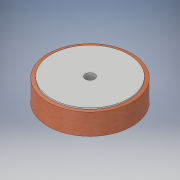
# Autodesk Inventor part: Rad
Saved by Autodesk Inventor 2017 (Build 210142000, 142)
## iProperties
Part Number: Rad
Material: Generisch
Document SubType Name: Modeling
Designer: Dima
Density: 1 g/cm^3
Appearance: Vorgabe
Author: Dima
Autodesk Inventor part; units mm, degrees
ref_plane "YZ Plane" through (0, 0, 0) normal (1, 0, 0) x (0, 1, 0)
ref_plane "XZ Plane" through (0, 0, 0) normal (0, 1, 0) x (-1, 0, 0)
ref_plane "XY Plane" through (0, 0, 0) normal (0, 0, 1) x (1, 0, 0)
sketch "Skizze1" plane through (0, 0, 0) normal (0, 1, 0) x (-1, 0, 0)
  line L0 (4, 10) -> (33, 10)
  line L1 (33, 10) -> (33, 9)
  line L2 (33, 9) -> (31, 9)
  line L3 (31, 9) -> (31, -9)
  line L4 (31, -9) -> (33, -9)
  line L5 (33, -9) -> (33, -10)
  line L6 (33, -10) -> (11.5, -10)
  line L7 (11.5, -10) -> (11.5, -5.5)
  line L8 (11.5, -5.5) -> (4, -5.5)
  line L9 (4, -5.5) -> (4, 10)
  line L10 (0, -14) -> (0, 14) construction
  line L11 (39.6, 0) -> (-6.6, 0) construction
  point P0 (0, 0)
  point P1 (31, 0)
  dimension "d0" = 4
  dimension "d1" = 2
  dimension "d2" = 33
  dimension "d3" = 18
  dimension "d4" = 20
  dimension "d5" = 4.5
  dimension "d6" = 11.5
  constraints: 20 end point, 8 perpendicular, 2 point on line, 1 horizontal, 1 horizontal alignment, 1 midpoint, 1 symmetric about line
  measures "d0" distance between parallel lines of L10 L9
  measures "d1" distance of L3.end L4.end
  measures "d2" distance from line of L10 L5.end
  measures "d3" distance of L2.end L3.end
  measures "d4" distance of L0.end L5.end
  measures "d5" distance of L6.end L7.end
  measures "d6" distance from line of L10 L6.end
revolve "Umdrehung1" add sketch "Skizze1" angle 360 about axis through (0, 0, -10) along (0, 0, 1)
sketch "Skizze2" plane through (0, 0, 0) normal (1, 0, 0) x (0, 1, 0)
  line L0 (-33, -9) -> (33, -9) construction
  line L1 (31, 9) -> (31, -9) construction
  line L2 (-33, 9) -> (33, 9) construction
  line L3 (36, -9) -> (31, -9)
  line L4 (31, -9) -> (31, 9)
  line L5 (31, 9) -> (36, 9)
  line L6 (36, 9) -> (36, -9)
  line L7 (0, -14) -> (0, 14) projected
  point P0 (0, 0)
  dimension "d8" = 5
  constraints: 8 end point, 2 parallel, 1 horizontal, 1 perpendicular
  measures "d8" distance of L3.start L1.end
revolve "Umdrehung2" add sketch "Skizze2" angle 360 about axis through (0, 0, -10) along (0, 0, 1) separate body
